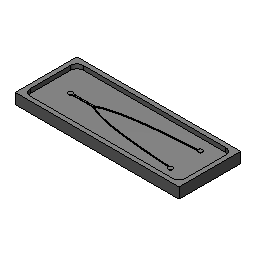
Microlfuidic Splitter 5 Speed Toolpaths (Autodesk Fusion 360 design; units mm, degrees)
Autodesk Fusion 360 part; units mm, degrees
sketch "Sketch1" plane through (0, 0, 0) normal (0, 0, 1) x (1, 0, 0)
  line L0 (0, 0) -> (60, 0)
  line L1 (60, 0) -> (60, 20)
  line L2 (60, 20) -> (0, 20)
  line L3 (0, 20) -> (0, 0)
  line L4 (3.9639, 10.3) -> (13.954, 10.3)
  line L5 (13.954, 9.7) -> (3.9639, 9.7)
  line L6 (40, 13.5098) -> (40, 13.5)
  line L7 (13.954, 13.5) -> (13.954, 13.5098)
  line L8 (14.111, 10.0441) -> (14.111, 9.9559)
  spline S0 degree 3 poles (14.111, 10.0441) (16.3875, 11.3257) (20.0042, 12.4691) (25.1292, 13.4206) (31.0485, 14.5196) (38.9488, 15.373) (48.0292, 16.0768) (50.6119, 16.277) (53.2926, 16.4648) (56.0667, 16.6409) knots 0.000559 0.000559 0.000559 0.000559 0.397017 0.397017 0.397017 0.854923 0.854923 0.854923 0.985161 0.985161 0.985161 0.985161
  spline S1 degree 3 poles (57, 16.6994) (57.0062, 16.6998) (57.0124, 16.7002) (57.0186, 16.7006) knots 0.999712 0.999712 0.999712 0.999712 1 1 1 1
  spline S2 degree 5 poles (13.954, 10.3) (14.3058, 10.4984) (15.0599, 10.8889) (16.3424, 11.4555) (18.3604, 12.172) (21.4224, 12.9992) (25.0503, 13.7549) (29.2412, 14.4393) (33.9504, 15.0581) (39.1215, 15.6184) (44.5257, 16.1114) (49.0827, 16.4687) (52.5912, 16.7157) (54.9227, 16.8688) (56.002, 16.9374) knots 0 0 0 0 0 0 0.1 0.2 0.3 0.4 0.5 0.6 0.7 0.8 0.9 0.984445 0.984445 0.984445 0.984445 0.984445 0.984445
  line L9 (50.6246, 16.5957) -> (61.3794, 17.279)
  arc A0 (56.0667, 16.6409) -> (56.002, 16.9374) centre (57, 17) ccw
  line L10 (57, 16.6994) -> (57, 17)
  spline S3 degree 3 poles (14.111, 9.9559) (16.3875, 8.6743) (20.0042, 7.5309) (25.1292, 6.5794) (31.0485, 5.4804) (38.9488, 4.627) (48.0292, 3.9232) (50.6119, 3.723) (53.2926, 3.5352) (56.0667, 3.3591) knots 0.000559 0.000559 0.000559 0.000559 0.397017 0.397017 0.397017 0.854923 0.854923 0.854923 0.985161 0.985161 0.985161 0.985161
  spline S4 degree 5 poles (13.954, 9.7) (14.3058, 9.5016) (15.0599, 9.1111) (16.3424, 8.5445) (18.3604, 7.828) (21.4224, 7.0008) (25.0503, 6.2451) (29.2412, 5.5607) (33.9504, 4.9419) (39.1215, 4.3816) (44.5257, 3.8886) (49.0827, 3.5313) (52.5912, 3.2843) (54.9227, 3.1312) (56.002, 3.0626) knots 0 0 0 0 0 0 0.1 0.2 0.3 0.4 0.5 0.6 0.7 0.8 0.9 0.984445 0.984445 0.984445 0.984445 0.984445 0.984445
  line L11 (11.2725, 8.7875) -> (16.6355, 11.8125)
  line L12 (11.2725, 11.2125) -> (16.6355, 8.1875)
  line L13 (50.6246, 3.4043) -> (61.3794, 2.721)
  arc A1 (56.002, 3.0626) -> (56.0667, 3.3591) centre (57, 3) ccw
  arc A2 (3.9639, 10.3) -> (3.9639, 9.7) centre (3.01, 10) ccw
  point P0 (23.9539, 13.5)
  point P1 (23.9539, 6.5)
  dimension "d1" = 60
  dimension "d2" = 20
  dimension "d6" = 2
  constraint horizontal L0
  constraint vertical L1
  constraint horizontal L2
  constraint vertical L3
  constraint coincident L0.start L3.end
  constraint coincident A0.centre L10.end
  constraint horizontal L4
  constraint horizontal L5
  constraint vertical L8
  constraint midpoint S2.end L9
  constraint midpoint L4.end L11
  measures "d1" distance of L0.start L0.end
  measures "d2" distance of L0.start L2.end
  measures "d6" diameter of A0
extrude "Extrude1" add sketch "Sketch1" along normal blind 3.3 contours L13 A1 | L8 S0 S2 L9 A0 S3 S4 L11 L12 L13 A1 | L9 A0 | L5 L11 L12 | L4 L11 L12 | L4 L5 L11 L12 A2 makes body 1
extrude "Extrude2" add sketch "Sketch1" along normal blind 3 contours L0 L1 L2 L3 L4 L5 S2 L9 A0 S4 L13 A1 A2 | L1 L8 S0 L9 A0 S3 L13 A1 bodies 1
sketch "Sketch2" plane through (0, 0, 0) normal (0, 0, -1) x (1, 0, 0)
  line L0 (0, 0) -> (0, -20)
  line L1 (0, -20) -> (60, -20)
  line L2 (60, -20) -> (60, 0)
  line L3 (60, 0) -> (0, 0)
  line L4 (-2.5, 2.5) -> (62.5, 2.5)
  line L5 (62.5, 2.5) -> (62.5, -22.5)
  line L6 (62.5, -22.5) -> (-2.5, -22.5)
  line L7 (-2.5, -22.5) -> (-2.5, 2.5)
  dimension "d16" = 65
  dimension "d17" = 25
  constraint horizontal L4
  constraint vertical L5
  constraint horizontal L6
  constraint vertical L7
  measures "d16" distance of L4.start L4.end
  measures "d17" distance of L4.start L6.end
extrude "Extrude3" add sketch "Sketch2" along normal blind 2 separate body makes body 2
extrude "Extrude4" add 1 faces at (62.5, 5.8333, -0.6667) along direction (1, 0, 0) blind 1 on bodies 2 bodies 2
extrude "Extrude5" add 1 faces at (41.5, 22.5, -1.3333) along direction (0, 1, 0) blind 2 on bodies 2 bodies 2
extrude "Extrude6" add 1 faces at (63.5, 15.5, -1.3333) along direction (1, 0, 0) blind 1 on bodies 2 bodies 2
extrude "Extrude7" add 1 faces at (42.1667, -2.5, -1.3333) along direction (0, -1, 0) blind 2 on bodies 2 bodies 2
extrude "Extrude8" add 1 faces at (-2.5, 5.1667, -1.3333) along direction (-1, 0, 0) blind 2 on bodies 2 bodies 2
sketch "Sketch3" plane through (0, 0, 0) normal (0, 0, 1) x (1, 0, 0)
  line L0 (-4.05, -19.95) -> (64.1, -19.95)
  line L1 (64.1, -19.95) -> (64.1, -40.1)
  line L2 (64.1, -40.1) -> (-4.05, -40.1)
  line L3 (-4.05, -40.1) -> (-4.05, -19.95)
  line L4 (-6, -18) -> (66.05, -18)
  line L5 (66.05, -18) -> (66.05, -42.05)
  line L6 (66.05, -42.05) -> (-6, -42.05)
  line L7 (-6, -42.05) -> (-6, -18)
  constraint horizontal L0
  constraint vertical L1
  constraint horizontal L2
  constraint vertical L3
  constraint horizontal L4
  constraint vertical L5
  constraint horizontal L6
  constraint vertical L7
combine "Combine1" operation add target body 1 tool bodies 2
copy_body "Body->Comp1" bodies 1 removing the originals makes body 3 in component "splitter"
extrude "Extrude1'" add 1 faces at (20, 13.3333, 0) along direction (0, 0, -1) blind 2 on bodies 3 bodies 3 in component "splitter"
extrude "Extrude2'" add 1 faces at (18.5, 5.1667, -2) along direction (0, 0, -1) blind 5 on bodies 3 bodies 3 in component "splitter"
move_face "OffsetFaces1" offset 4 1 faces at (64.5, 5.1667, -2.3333) on bodies 3 in component "splitter"
move_face "OffsetFaces2" offset 4 1 faces at (60, 6.6667, 1) on bodies 3 in component "splitter"
move_face "OffsetFaces3" offset 4 2 faces at (0, 13.3333, 1) (-4.5, 14.8333, -4.6667) on bodies 3 in component "splitter"
extrude "Extrude3'" add 1 faces at (18.6667, -3, 0) along direction (0, 0, 1) blind 5 on bodies 3 bodies 3 in component "splitter"
extrude "Extrude4'" cut 1 faces at (42.8333, 14.8333, -7) along direction (0, 0, 1) blind 8 on bodies 3 bodies 3 in component "splitter"
extrude "Extrude5'" add 1 faces at (42.8333, 14.8333, 1) along direction (0, 0, -1) blind 1 on bodies 3 bodies 3 in component "splitter"
move_face "OffsetFaces4" offset -2.5 2 faces at (41.3333, 20, 3.6667) (41.3333, 0, 3.6667) on bodies 3 in component "splitter"
move_face "OffsetFaces5" offset -2.5 2 faces at (64, 5.8333, 4.3333) (-4, 14.1667, 3.6667) on bodies 3 in component "splitter"
fillet "Fillet1" radius 3 4 edges at (-6.5, 22.5, 4) (66.5, 22.5, 4) (66.5, -2.5, 4) (-6.5, -2.5, 4) on bodies 3 in component "splitter"
ref_plane "WorkPlane1" through (7.5, 10, 2.5) normal (1, 0, 0) x (0, 0, -1)
ref_plane "WorkPlane2" through (48.5, 10, 2.5) normal (1, 0, 0) x (0, 0, -1)
component "splitter" placed x (1, 0, 0) y (0, 1, 0) z (0, 0, 1) at (0, 0, 0)
named bodies: "splitter"
